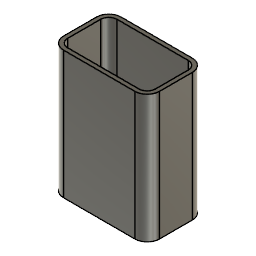
▢-75X45X3.2 (Autodesk Fusion 360 design; units mm, degrees)
Autodesk Fusion 360 part; units mm, degrees
sketch "スケッチ1" plane through (0, 0, 0) normal (0, 0, 1) x (1, 0, 0)
  line L0 (107.8352, 303.5645) -> (163.6352, 303.5645)
  line L1 (107.8352, 306.7645) -> (163.6352, 306.7645)
  line L2 (163.6352, 348.5645) -> (107.8352, 348.5645)
  line L3 (163.6352, 345.3645) -> (107.8352, 345.3645)
  line L4 (98.2352, 338.9645) -> (98.2352, 313.1645)
  line L5 (101.4352, 338.9645) -> (101.4352, 313.1645)
  arc A0 (98.2352, 313.1645) -> (107.8352, 303.5645) centre (107.8352, 313.1645) ccw
  arc A1 (101.4352, 313.1645) -> (107.8352, 306.7645) centre (107.8352, 313.1645) ccw
  arc A2 (107.8352, 348.5645) -> (98.2352, 338.9645) centre (107.8352, 338.9645) ccw
  arc A3 (107.8352, 345.3645) -> (101.4352, 338.9645) centre (107.8352, 338.9645) ccw
  line L6 (173.2352, 313.1645) -> (173.2352, 338.9645)
  line L7 (170.0352, 313.1645) -> (170.0352, 338.9645)
  arc A4 (163.6352, 303.5645) -> (173.2352, 313.1645) centre (163.6352, 313.1645) ccw
  arc A5 (163.6352, 306.7645) -> (170.0352, 313.1645) centre (163.6352, 313.1645) ccw
  arc A6 (173.2352, 338.9645) -> (163.6352, 348.5645) centre (163.6352, 338.9645) ccw
  arc A7 (170.0352, 338.9645) -> (163.6352, 345.3645) centre (163.6352, 338.9645) ccw
  point P0 (135.7352, 326.0645)
extrude "押し出し1" add sketch "スケッチ1" along normal blind 100
